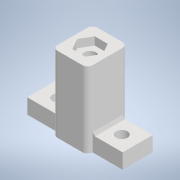
# Autodesk Inventor part: Hopper Rest Metric Wide
Saved by Autodesk Inventor 2022 (Build 260153000, 153)
## iProperties
Created: 2021-06-02
Part Number: Hopper Rest Metric Wide
Material: Generic
Document SubType Name: Modeling
Designer: John
Density: 1 g/cm^3
Appearance: Default
Author: John
Autodesk Inventor part; units mm, degrees
ref_plane "YZ Plane" through (0, 0, 0) normal (1, 0, 0) x (0, 1, 0)
ref_plane "XZ Plane" through (0, 0, 0) normal (0, 1, 0) x (-1, 0, 0)
ref_plane "XY Plane" through (0, 0, 0) normal (0, 0, 1) x (1, 0, 0)
sketch "Sketch1" plane through (0, 0, 0) normal (0, 1, 0) x (-1, 0, 0)
  line L0 (0, 0) -> (0, -12)
  line L1 (0, -12) -> (38.1, -12)
  line L2 (38.1, -12) -> (38.1, 0)
  line L3 (38.1, 0) -> (0, 0)
  circle A0 centre (6.35, -6) radius 1.6256
  circle A1 centre (31.75, -6) radius 1.6256
  point P0 (0, -6)
  dimension "d0" = 3.2512
  dimension "d1" = 3.2512
  dimension "d3" = 0
  dimension "d4" = 12
  dimension "d6" = 38.1
  dimension "d37" = 6.35
  dimension "d38" = 6.35
  constraints: 8 end point, 3 perpendicular, 2 centre point, 1 horizontal alignment, 1 midpoint, 1 vertical
  measures "d0" diameter of A0
  measures "d1" diameter of A1
  measures "d3" vertical distance of A0.centre A1.centre
  measures "d4" distance between parallel lines of L1 L3
  measures "d6" distance between parallel lines of L0 L2
  measures "d37" distance from line of L2 A1.centre
  measures "d38" distance from line of L0 A0.centre
extrude "Extrusion1" add sketch "Sketch1" along normal blind 6 contours L3 L2 L1 L0 | A0 | A1
sketch "Sketch3" plane through (0, 6, 0) normal (0, 1, 0) x (1, 0, 0)
  line L0 (-14.05, 0) -> (-24.05, 0)
  line L1 (-24.05, 0) -> (-24.05, 12)
  line L2 (-24.05, 12) -> (-14.05, 12)
  line L3 (-14.05, 12) -> (-14.05, 0)
  line L4 (-38.1, 0) -> (0, 0) projected
  line L5 (0, 0) -> (0, 12) projected
  line L6 (0, 12) -> (-38.1, 12) projected
  point P0 (-19.05, 12)
  point P1 (-19.05, 12)
  point P2 (-19.05, 12)
  dimension "d12" = 10
  dimension "d14" = 0
  constraints: 8 end point, 3 midpoint, 2 coincident, 2 parallel, 1 horizontal, 1 perpendicular
  measures "d12" distance of L1.end L2.end
  measures "d14" distance between parallel lines of L4 L0
extrude "Extrusion3" add sketch "Sketch3" along normal blind 24.13 contours L0 L1 L2 L3
chamfer "Chamfer1" distance 3 angle 45 2 edges at (-14.05, 6, -6) (-24.05, 6, -6)
sketch "Sketch5" plane through (0, 30.13, 0) normal (0, 1, 0) x (1, 0, 0)
  line L0 (-14.05, 12) -> (-24.05, 12) projected
  line L1 (-14.05, 0) -> (-14.05, 12) projected
  point P0 (0, 0)
  point P1 (-19.05, 6)
  point P2 (-19.05, 12)
  point P3 (-14.05, 6)
  constraints: 2 midpoint, 1 horizontal alignment, 1 vertical alignment
hole "Hole1" at (-19.05, 30.13, -6) direction (0, -1, 0) diameter 4.7 end through all clearance for "Flat Head Machine Screw" size "M4" standard "Ansi Metric M Profile"
hole "Hole2" at (-6.35, 0, -6) at (-31.75, 0, -6) direction (0, 1, 0) diameter 4.5 end through all clearance for "Flat Head Machine Screw" size "M4" standard "Ansi Metric M Profile"
sketch "Sketch7" plane through (0, 30.13, 0) normal (0, 1, 0) x (1, 0, 0)
  line L0 (-14.05, 12) -> (-24.05, 12) projected
  line L1 (-24.05, 12) -> (-24.05, 14)
  line L2 (-24.05, 14) -> (-14.05, 14)
  line L3 (-11.05, 12) -> (-14.05, 12) projected
  line L4 (-24.05, 12) -> (-14.05, 12)
  line L5 (-14.05, 0) -> (-14.05, 12) projected
  line L6 (-14.05, 0) -> (-14.05, -2)
  line L7 (-14.05, -2) -> (-24.05, -2)
  line L8 (-24.05, 0) -> (-14.05, 0) projected
  line L9 (-24.05, -2) -> (-24.05, 0)
  line L10 (-24.05, 0) -> (-14.05, 0)
  line L11 (-24.05, 14) -> (-26.05, 14)
  line L12 (-26.05, 14) -> (-26.05, -2)
  line L13 (-26.05, -2) -> (-24.05, -2)
  line L14 (-24.05, -2) -> (-24.05, 14)
  line L15 (-14.05, -2) -> (-12.05, -2)
  line L16 (-12.05, -2) -> (-12.05, 14)
  line L17 (-12.05, 14) -> (-14.05, 14)
  line L18 (-14.05, 12) -> (-14.05, -2)
  point P0 (0, 0)
  point P1 (-12.05, 12)
  point P2 (-24.05, 0)
  point P3 (-25.05, -2)
  dimension "d41" = 2
  dimension "d42" = 2
  dimension "d43" = 2
  dimension "d44" = 2
  constraints: 30 end point, 5 perpendicular, 4 parallel, 3 horizontal, 2 point on line, 2 vertical, 1 collinear, 1 horizontal alignment, 1 midpoint
  measures "d41" distance of L0.end L1.end
  measures "d42" distance of L5.start L6.end
  measures "d43" distance of L13.end L12.end
  measures "d44" distance of L17.end L16.end
extrude "Extrusion6" add sketch "Sketch7" against normal up to surface (30.13 mm away) contours L0 L1 L2 L17 L16 L3 | L3 L16 L15 L6 L5 | L14 L9 L13 L12 L11 L1 | L6 L7 L9 L8
sketch "Sketch6" plane through (0, 30.13, 0) normal (0, 1, 0) x (1, 0, 0)
  line L0 (-17.0293, 9.5) -> (-16.0189, 7.75) projected
  line L1 (-16.0189, 7.75) -> (-15.0085, 6) projected
  line L2 (-15.0085, 6) -> (-16.0189, 4.25) projected
  line L3 (-16.0189, 4.25) -> (-17.0293, 2.5) projected
  line L4 (-17.0293, 2.5) -> (-19.05, 2.5) projected
  line L5 (-19.05, 2.5) -> (-21.0707, 2.5) projected
  line L6 (-21.0707, 2.5) -> (-22.0811, 4.25) projected
  line L7 (-22.0811, 4.25) -> (-23.0915, 6) projected
  line L8 (-23.0915, 6) -> (-22.0811, 7.75) projected
  line L9 (-22.0811, 7.75) -> (-21.0707, 9.5) projected
  line L10 (-21.0707, 9.5) -> (-19.05, 9.5) projected
  line L11 (-19.05, 9.5) -> (-17.0293, 9.5) projected
  line L12 (-19.05, 10.3656) -> (-21.5705, 10.3656) projected
  line L13 (-16.5295, 10.3656) -> (-19.05, 10.3656) projected
  line L14 (-15.2693, 8.1828) -> (-16.5295, 10.3656) projected
  line L15 (-14.009, 6) -> (-15.2693, 8.1828) projected
  line L16 (-15.2693, 3.8172) -> (-14.009, 6) projected
  line L17 (-16.5295, 1.6344) -> (-15.2693, 3.8172) projected
  line L18 (-19.05, 1.6344) -> (-16.5295, 1.6344) projected
  line L19 (-21.5705, 1.6344) -> (-19.05, 1.6344) projected
  line L20 (-22.8307, 3.8172) -> (-21.5705, 1.6344) projected
  line L21 (-24.091, 6) -> (-22.8307, 3.8172) projected
  line L22 (-22.8307, 8.1828) -> (-24.091, 6) projected
  line L23 (-21.5705, 10.3656) -> (-22.8307, 8.1828) projected
  line L24 (-21.6282, 10.4656) -> (-16.4718, 10.4656)
  line L25 (-16.4718, 10.4656) -> (-13.8935, 6)
  line L26 (-13.8935, 6) -> (-16.4718, 1.5344)
  line L27 (-16.4718, 1.5344) -> (-21.6282, 1.5344)
  line L28 (-21.6282, 1.5344) -> (-24.2065, 6)
  line L29 (-24.2065, 6) -> (-21.6282, 10.4656)
  point P0 (0, 0)
  dimension "d50" = 0.1
  dimension "d51" = 0.1
  dimension "d52" = 0.1
  dimension "d53" = 0.1
  dimension "d54" = 0.1
  dimension "d55" = 0.1
  constraints: 12 end point, 5 parallel, 1 horizontal
  measures "d50" distance between parallel lines of L12 L24
  measures "d51" distance between parallel lines of L18 L27
  measures "d52" distance between parallel lines of L21 L28
  measures "d53" distance between parallel lines of L15 L25
  measures "d54" distance between parallel lines of L23 L29
  measures "d55" distance between parallel lines of L16 L26
extrude "Extrusion5" cut sketch "Sketch6" against normal blind 3.2 contours L0 L1 L2 L3 L4 L5 L6 L7 L8 L9 L10 L11 | L13 L14 L15 L16 L17 L18 L19 L20 L21 L22 L23 L12 | L24 L25 L26 L27 L28 L29
fillet "Fillet1" radius 2 4 edges at (-12.05, 15.065, -14) (-26.05, 15.065, -14) (-26.05, 15.065, 2) (-12.05, 15.065, 2)
body "Solid1"
